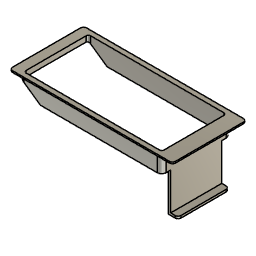
Poop Bucket Dowel (Autodesk Fusion 360 design; units mm, degrees)
Autodesk Fusion 360 part; units mm, degrees
sketch "Sketch2" plane through (0, 0, 0) normal (0, 0, -1) x (1, 0, 0)
  line L0 (0, 0) -> (0, -80)
  line L1 (0, -80) -> (120, -80)
  line L2 (120, -80) -> (120, 0)
  line L3 (120, 0) -> (0, 0)
  line L4 (18, -18.25) -> (108, -18.25)
  line L5 (109.5, -19.75) -> (109.5, -60.25)
  line L6 (108, -61.75) -> (18, -61.75)
  line L7 (16.5, -60.25) -> (16.5, -19.75)
  arc A0 (18, -18.25) -> (16.5, -19.75) centre (18, -19.75) ccw
  arc A1 (16.5, -60.25) -> (18, -61.75) centre (18, -60.25) ccw
  arc A2 (109.5, -19.75) -> (108, -18.25) centre (108, -19.75) ccw
  arc A3 (108, -61.75) -> (109.5, -60.25) centre (108, -60.25) ccw
  point P0 (16.5, -18.25)
  point P1 (109.5, -18.25)
  point P2 (16.5, -61.75)
  dimension "d8" = 93
  dimension "d9" = 43.5
  dimension "d10" = 18.25
  dimension "d11" = 18.25
  dimension "d12" = 16.5
  dimension "d15" = 1.5
  dimension "d16" = 1.5
  constraint horizontal L4
  constraint vertical L5
  constraint horizontal L6
  constraint vertical L7
  constraint coincident P0 L4
  constraint coincident P0 L7
  constraint tangent L4 A0
  constraint tangent L7 A0
  constraint coincident P2 L6
  constraint coincident P2 L7
  constraint tangent L6 A1
  constraint tangent L7 A1
  constraint coincident P1 L4
  constraint coincident P1 L5
  constraint tangent L4 A2
  constraint tangent L5 A2
  constraint equal A1 A2
  constraint tangent L5 A3
  constraint tangent L6 A3
  constraint equal A1 A3
  measures "d8" distance of P0 P1
  measures "d9" distance of P0 P2
  measures "d10" distance of L3 L4
  measures "d11" distance of L1 L6
  measures "d12" distance of L0 L7
  measures "d15" radius of A0
  measures "d16" radius of A1
sketch "Sketch3" plane through (0, 0, 0) normal (0, 0, -1) x (1, 0, 0)
  line L0 (18, -18.25) -> (108, -18.25)
  arc A0 (109.5, -19.75) -> (108, -18.25) centre (108, -19.75) ccw
  line L1 (109.5, -19.75) -> (109.5, -60.25)
  arc A1 (108, -61.75) -> (109.5, -60.25) centre (108, -60.25) ccw
  line L2 (108, -61.75) -> (18, -61.75)
  arc A2 (16.5, -60.25) -> (18, -61.75) centre (18, -60.25) ccw
  line L3 (16.5, -60.25) -> (16.5, -19.75)
  arc A3 (18, -18.25) -> (16.5, -19.75) centre (18, -19.75) ccw
  line L4 (0, 0) -> (0, -80)
  line L5 (0, -80) -> (120, -80)
  line L6 (120, -80) -> (120, 0)
  line L7 (120, 0) -> (0, 0)
  arc A4 (111, -19.75) -> (108, -16.75) centre (108, -19.75) ccw
  line L8 (18, -16.75) -> (108, -16.75)
  arc A5 (18, -16.75) -> (15, -19.75) centre (18, -19.75) ccw
  line L9 (15, -60.25) -> (15, -19.75)
  arc A6 (15, -60.25) -> (18, -63.25) centre (18, -60.25) ccw
  line L10 (108, -63.25) -> (18, -63.25)
  arc A7 (108, -63.25) -> (111, -60.25) centre (108, -60.25) ccw
  line L11 (111, -19.75) -> (111, -60.25)
  dimension "d17" = -1.5
extrude "Extrude3" add sketch "Sketch3" along normal blind 11.5 contours A4 L8 A5 L9 A6 L10 A7 L11
sketch "Sketch4" plane through (0, 16.75, 0) normal (0, -1, 0) x (1, 0, 0)
  line L0 (18, 0) -> (18, -11.5)
  line L1 (18, -11.5) -> (108, -11.5)
  line L2 (108, -11.5) -> (108, 0)
  line L3 (15, 0) -> (15, -1.6) construction
  line L4 (15, -1.6) -> (29.14, -11.5)
  line L5 (15, 0) -> (15, -11.5)
  line L6 (29.14, -11.5) -> (15, -11.5)
  line L7 (15, -1.6) -> (15, -11.5)
  line L8 (108, 0) -> (18, 0)
  point P0 (15, -11.5)
  dimension "d20" = 1.6
  dimension "d21" = 14.14
  constraint vertical L3
  constraint coincident L1 L4.end
  constraint coincident L3.end L5
  constraint coincident P0 L5.end
  measures "d20" distance of L3.start L3.end
  measures "d21" distance of L4.end P0
extrude "Extrude4" cut sketch "Sketch4" against normal up to surface (46.5 mm away) contours L0 L1 L4 L6 | L0 L4 L5 L6 L7
sketch "Sketch5" plane through (0, 0, -11.5) normal (0, 0, -1) x (1, 0, 0)
  line L0 (29.14, -63.25) -> (108, -63.25)
  arc A0 (108, -63.25) -> (111, -60.25) centre (108, -60.25) ccw
  line L1 (111, -60.25) -> (111, -19.75)
  arc A1 (111, -19.75) -> (108, -16.75) centre (108, -19.75) ccw
  line L2 (108, -16.75) -> (29.14, -16.75)
  line L3 (29.14, -18.25) -> (108, -18.25)
  arc A2 (109.5, -19.75) -> (108, -18.25) centre (108, -19.75) ccw
  line L4 (109.5, -19.75) -> (109.5, -60.25)
  arc A3 (108, -61.75) -> (109.5, -60.25) centre (108, -60.25) ccw
  line L5 (108, -61.75) -> (29.14, -61.75)
  line L6 (109.5, -22.75) -> (111, -22.75)
  line L7 (111, -22.75) -> (111, -57.25)
  line L8 (111, -57.25) -> (109.5, -57.25)
  line L9 (109.5, -57.25) -> (109.5, -22.75)
  line L10 (29.14, -16.75) -> (29.14, -18.25)
  line L11 (29.14, -61.75) -> (29.14, -63.25)
  dimension "d26" = 1.5
  dimension "d27" = 34.5
  dimension "d28" = 4.5
  dimension "d29" = 4.5
  constraint horizontal L6
  constraint vertical L7
  constraint horizontal L8
  constraint vertical L9
  constraint coincident L4 L6.start
  measures "d26" distance of L6.start L6.end
  measures "d27" distance of L6.start L8.end
  measures "d28" distance of L3 L6.start
  measures "d29" distance of L5 L8.end
extrude "Extrude5" add sketch "Sketch5" along normal blind 26.5 contours L1 L4 L6 L7 L8 L9
sketch "Sketch6" plane through (111, 0, 0) normal (1, 0, 0) x (0, 1, 0)
  line L0 (19.75, 0) -> (19.75, -11.5)
  line L1 (19.75, -11.5) -> (22.75, -11.5)
  line L2 (22.75, -11.5) -> (22.75, -38)
  line L3 (22.75, -38) -> (57.25, -38)
  line L4 (57.25, -38) -> (57.25, -11.5)
  line L5 (57.25, -11.5) -> (60.25, -11.5)
  line L6 (60.25, -11.5) -> (60.25, 0)
  line L7 (22.75, -38) -> (57.25, -38)
  line L8 (57.25, -38) -> (57.25, -36.5)
  line L9 (57.25, -36.5) -> (22.75, -36.5)
  line L10 (22.75, -36.5) -> (22.75, -38)
  line L11 (60.25, 0) -> (19.75, 0)
  dimension "d34" = 34.5
  dimension "d35" = 1.5
  constraint horizontal L7
  constraint vertical L8
  constraint horizontal L9
  constraint vertical L10
  constraint coincident L2.end L3.start
  measures "d34" distance of L2.end L3.end
  measures "d35" distance of L2.end L9.end
extrude "Extrude6" add sketch "Sketch6" along normal blind 5 contours L2 L3 L4 L7 L8 L9 L10
fillet "Fillet4" radius 2 2 edges at (116, 57.25, -37.25) (116, 22.75, -37.25)
sketch "Sketch7" plane through (0, 0, 0) normal (0, 0, 1) x (1, 0, 0)
  line L0 (120, 65) -> (10, 65)
  line L1 (10, 65) -> (10, 15)
  line L2 (10, 15) -> (120, 15)
  line L3 (120, 15) -> (120, 65)
  constraint horizontal L0
  constraint vertical L1
  constraint horizontal L2
  constraint vertical L3
extrude "Extrude7" add sketch "Sketch7" along normal blind 1
extrude "Extrude8" cut 1 faces at (78, 32.75, 0) along direction (0, 0, 1) up to surface (1 mm away)
fillet "Fillet5" radius 2 4 edges at (10, 15, 0.5) (120, 15, 0.5) (120, 65, 0.5) (10, 65, 0.5)
equation "d10 = d11"
equation "d28 = d29"
